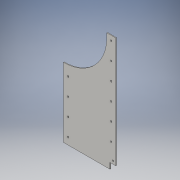
# Autodesk Inventor part: LauncherSidePlateRev2
Saved by Autodesk Inventor 2016 (Build 200138000, 138)
## iProperties
Created: 2017-01-21
Part Number: LauncherSidePlateRev2
Material: Generic
Document SubType Name: Modeling
Designer: madsenn
Density: 1 g/cm^3
Appearance: Default
Author: madsenn
Autodesk Inventor part; units mm, degrees
ref_plane "YZ Plane" through (0, 0, 0) normal (1, 0, 0) x (0, 1, 0)
ref_plane "XZ Plane" through (0, 0, 0) normal (0, 1, 0) x (-1, 0, 0)
ref_plane "XY Plane" through (0, 0, 0) normal (0, 0, 1) x (1, 0, 0)
sketch "Sketch1" plane through (0, 0, 0) normal (0, 0, 1) x (1, 0, 0)
  line L0 (229.6952, -414.7737) -> (228.902, -414.7737)
  line L1 (202.9458, -491.49) -> (202.9458, -465.836)
  line L2 (202.9458, -465.836) -> (228.5998, -465.836)
  line L3 (202.9458, -491.49) -> (-0.0002, -491.49)
  line L4 (-0.0002, -491.49) -> (-0.0002, -189.4332)
  arc A0 (-0.0002, -189.4332) -> (188.7124, 16.51) centre (0, 0) ccw
  line L5 (0, 0) -> (188.7124, 16.51) construction
  line L6 (0, 0) -> (-0.0002, -189.4332) construction
  line L7 (228.5998, -465.836) -> (228.5998, 16.51)
  line L8 (228.5998, 16.51) -> (188.7124, 16.51)
  circle A1 centre (20.5738, -232.664) radius 3.5687
  circle A2 centre (20.5738, -308.864) radius 3.5687
  circle A3 centre (20.5738, -385.064) radius 3.5687
  circle A4 centre (20.5738, -461.264) radius 3.5687
  circle A5 centre (215.8998, -453.136) radius 3.5687
  circle A6 centre (208.0258, -385.064) radius 3.5687
  circle A7 centre (208.0258, -308.864) radius 3.5687
  circle A8 centre (208.0258, -232.664) radius 3.5687
  circle A9 centre (208.0301, -156.464) radius 3.5687
  circle A10 centre (208.0258, -80.264) radius 3.5687
  circle A11 centre (208.0258, -4.064) radius 3.5687
  point P0 (208.0258, -461.264)
  dimension "d15" = 25.654
  dimension "d59" = 95
  dimension "d60" = 189.4332
  dimension "d61" = 508
  dimension "d62" = 76.2
  dimension "d63" = 76.2
  dimension "d65" = 20.5697
  dimension "d66" = 20.574
  dimension "d67" = 20.574
  dimension "d68" = 76.2
  dimension "d69" = 76.2
  dimension "d70" = 76.2
  dimension "d71" = 76.2
  dimension "d73" = 25.654
  dimension "d74" = 12.7
  dimension "d75" = 76.2
  dimension "d76" = 76.2
  dimension "d77" = 76.2
  dimension "d78" = 43.2308
  dimension "d79" = 20.574
  dimension "d80" = 20.574
  dimension "d81" = 20.574
  dimension "d82" = 20.574
  dimension "d85" = 7.1374
  dimension "d86" = 7.1374
  dimension "d87" = 7.1374
  dimension "d88" = 7.1374
  dimension "d89" = 7.1374
  dimension "d91" = 7.1374
  dimension "d92" = 7.1374
  dimension "d93" = 7.1374
  dimension "d94" = 7.1374
  dimension "d95" = 7.1374
  dimension "d96" = 7.1374
  dimension "d99" = 228.6
  dimension "d100" = 12.7
  dimension "d103" = 20.574
  dimension "d104" = 20.574
  dimension "d105" = 20.574
  dimension "d106" = 20.574
  dimension "d108" = 30.226
  dimension "d109" = 106.426
  constraints: 18 end point, 12 centre point, 12 coincident, 3 perpendicular, 2 horizontal, 2 point on circle, 1 parallel, 1 vertical
  measures "d15" distance of L2.end L1.end
  measures "d59" angle of L6 L5
  measures "d60" radius of A0
  measures "d61" distance between parallel lines of L3 L8
  measures "d62" distance of point (208.026, -80.264) point (208.026, -4.064)
  measures "d63" distance of point (208.03, -156.464) point (208.026, -80.264)
  measures "d65" distance from line of L7 point (208.03, -156.464)
  measures "d66" distance from line of L7 point (208.026, -232.664)
  measures "d67" distance from line of L8 point (208.026, -4.064)
  measures "d68" distance of point (208.026, -232.664) point (208.03, -156.464)
  measures "d69" distance of point (208.026, -232.664) point (208.026, -308.864)
  measures "d70" distance of point (208.026, -385.064) point (208.026, -308.864)
  measures "d71" distance of point (208.026, -461.264) point (208.026, -385.064)
  measures "d73" distance between parallel lines of L3 L2
  measures "d74" distance from line of L2 point (215.9, -453.136)
  measures "d75" distance of point (20.574, -308.864) point (20.574, -232.664)
  measures "d76" distance of point (20.574, -385.064) point (20.574, -308.864)
  measures "d77" distance of point (20.574, -461.264) point (20.574, -385.064)
  measures "d78" vertical distance of L4.end point (20.574, -232.664)
  measures "d79" distance from line of L4 point (20.574, -232.664)
  measures "d80" distance from line of L4 point (20.574, -308.864)
  measures "d81" distance from line of L4 point (20.574, -385.064)
  measures "d82" distance from line of L4 point (20.574, -461.264)
  measures "d85" diameter of A1
  measures "d86" diameter of A2
  measures "d87" diameter of A3
  measures "d88" diameter of A4
  measures "d89" diameter of A5
  measures "d91" diameter of A6
  measures "d92" diameter of A7
  measures "d93" diameter of A8
  measures "d94" diameter of A9
  measures "d95" diameter of A10
  measures "d96" diameter of A11
  measures "d99" distance between parallel lines of L7 L4
  measures "d100" distance from line of L7 point (215.9, -453.136)
  measures "d103" distance from line of L7 point (208.026, -308.864)
  measures "d104" distance from line of L7 point (208.026, -385.064)
  measures "d105" distance from line of L7 point (208.026, -461.264)
  measures "d106" distance from line of L7 point (208.026, -80.264)
  measures "d108" distance from line of L3 point (20.574, -461.264)
  measures "d109" distance from line of L3 point (208.026, -385.064)
extrude "Extrusion5" add sketch "Sketch1" along normal blind 3.175
body "Solid4"
